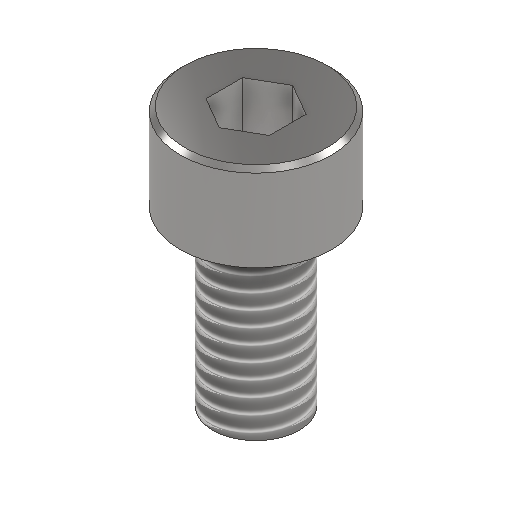
# Autodesk Inventor part: M4×8-VentedHexSocket
Saved by Autodesk Inventor 2026.2 (Build 302298000, 298)
## iProperties
Created: 2026-07-16
Part Number: M4×8-VentedHexSocket
Material: ステンレス鋼
Document SubType Name: Modeling
Designer: zetsu
Density: 8 g/cm^3
Appearance: 半つや出し
Author: zetsu
Autodesk Inventor part; units mm, degrees
ref_plane "YZ Plane" through (0, 0, 0) normal (1, 0, 0) x (0, 1, 0)
ref_plane "XZ Plane" through (0, 0, 0) normal (0, 1, 0) x (-1, 0, 0)
ref_plane "XY Plane" through (0, 0, 0) normal (0, 0, 1) x (1, 0, 0)
sketch "スケッチ1" plane through (0, 0, 0) normal (0, 1, 0) x (-1, 0, 0)
  circle A0 centre (0, 0) radius 2
  dimension "d0" = 4
  constraints: 1 centre point, 1 coincident
  measures "d0" diameter of A0
extrude "押し出し1" add sketch "スケッチ1" against normal blind 8
sketch "スケッチ2" plane through (0, 0, 0) normal (0, 1, 0) x (1, 0, 0)
  circle A0 centre (0, 0) radius 2 projected
  circle A1 centre (0, 0) radius 3.5
  dimension "d3" = 7
  constraints: 1 centre point, 1 coincident
  measures "d3" diameter of A1
extrude "押し出し2" add sketch "スケッチ2" along normal blind 4 contours A0 | A1
sketch "スケッチ3" plane through (0, 4, 0) normal (0, 1, 0) x (1, 0, 0)
  circle A0 centre (0, 0) radius 1.7 construction
  line L0 (0, 1.7) -> (-1.4722, 0.85)
  line L1 (-1.4722, 0.85) -> (-1.4722, -0.85)
  line L2 (-1.4722, -0.85) -> (0, -1.7)
  line L3 (0, -1.7) -> (1.4722, -0.85)
  line L4 (1.4722, -0.85) -> (1.4722, 0.85)
  line L5 (1.4722, 0.85) -> (0, 1.7)
  dimension "d6" = 3.4
  dimension "d9" = 360
  constraints: 12 end point, 2 point on circle, 1 centre point, 1 coincident, 19 other
  measures "d6" diameter of A0
extrude "押し出し3" cut sketch "スケッチ3" against normal blind 2.3
chamfer "面取り1" distance 0.2 angle 45 1 edges at (-3.5, 4, 0)
thread "ねじ1" size "M4x0.7" class "6g" standard "ANSI Metric M Profile" full length
sketch "スケッチ4" plane through (0, 1.7, 0) normal (0, 1, 0) x (1, 0, 0)
  circle A0 centre (0, 0) radius 0.5
  dimension "d18" = 1
  constraints: 1 centre point, 1 coincident
  measures "d18" diameter of A0
extrude "押し出し4" cut sketch "スケッチ4" against normal through all
